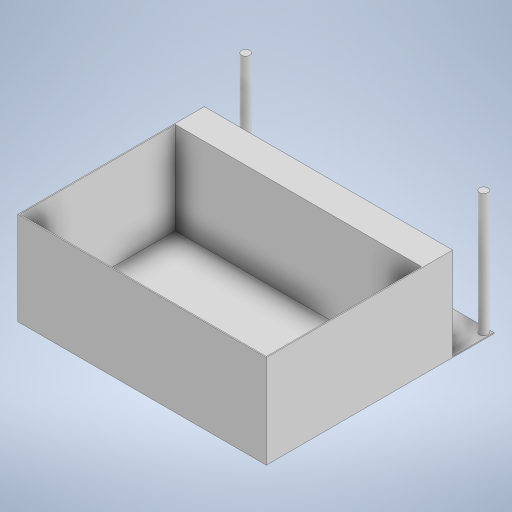
# Autodesk Inventor part: Distanced Top Bin
Saved by Autodesk Inventor 2024 (Build 280153000, 153)
## iProperties
Created: 2024-09-18
Part Number: Distanced Top Bin
Material: Generic
Document SubType Name: Modeling
Designer: srira
Density: 1 g/cm^3
Appearance: Default
Author: srira
Autodesk Inventor part; units mm, degrees
ref_plane "YZ Plane" through (0, 0, 0) normal (1, 0, 0) x (0, 1, 0)
ref_plane "XZ Plane" through (0, 0, 0) normal (0, 1, 0) x (-1, 0, 0)
ref_plane "XY Plane" through (0, 0, 0) normal (0, 0, 1) x (1, 0, 0)
sketch "Sketch1" plane through (0, 0, 0) normal (0, 1, 0) x (-1, 0, 0)
  line L0 (-600, 450) -> (600, 450)
  line L1 (600, 450) -> (600, -450)
  line L2 (600, -450) -> (-600, -450)
  line L3 (-600, -450) -> (-600, 450)
  line L4 (-600, 450) -> (600, -450) construction
  line L5 (600, 450) -> (-600, -450) construction
  line L6 (595, 445) -> (-595, 445)
  line L7 (-595, 445) -> (-595, -305)
  line L8 (-595, -305) -> (595, -305)
  line L9 (595, -305) -> (595, 445)
  point P0 (0, 0)
  dimension "d0" = 1200
  dimension "d1" = 900
  dimension "d2" = 1190
  dimension "d3" = 750
  constraints: 20 end point, 4 parallel, 2 horizontal, 2 midpoint, 2 perpendicular
  measures "d0" distance of L1.end L2.end
  measures "d1" distance of L0.end L1.end
  measures "d2" distance of L8.end L7.end
  measures "d3" distance of L7.end L6.end
extrude "Extrusion1" add sketch "Sketch1" along normal blind 450
ref_plane "Work Plane3" through (0, 0, 0) normal (0, 1, 0) x (1, 0, 0)
sketch "Sketch4" plane through (0, 0, 0) normal (0, 1, 0) x (1, 0, 0)
  line L0 (600, 450) -> (-600, 450) projected
  line L1 (-600, 450) -> (600, 450)
  line L2 (600, 450) -> (600, 650)
  line L3 (600, 650) -> (-600, 650)
  line L4 (-600, 650) -> (-600, 450)
  circle A0 centre (-575, 625) radius 20
  circle A1 centre (575, 625) radius 20
  point P0 (0, 0)
  dimension "d12" = 1200
  dimension "d13" = 200
  dimension "d14" = 40
  dimension "d15" = 40
  constraints: 8 end point, 2 centre point, 2 parallel, 1 horizontal, 1 perpendicular
  measures "d12" distance of L3.end L2.end
  measures "d13" distance of L2.end L1.end
  measures "d14" diameter of A0
  measures "d15" diameter of A1
extrude "Extrusion2" add sketch "Sketch4" along normal blind 600 contours A0 | A1
ref_plane "Work Plane6" through (0, 0, 0) normal (0, 1, 0) x (1, 0, 0)
sketch "Sketch5" plane through (0, 0, 0) normal (0, 1, 0) x (1, 0, 0)
  line L0 (-600, 450) -> (600, 450)
  line L1 (600, 450) -> (600, 650)
  line L2 (600, 650) -> (-600, 650)
  line L3 (-600, 650) -> (-600, 450)
  point P0 (0, 0)
  dimension "d18" = 1200
  dimension "d19" = 200
  constraints: 8 end point, 2 parallel, 1 horizontal, 1 perpendicular
  measures "d18" distance of L2.end L1.end
  measures "d19" distance of L1.end L0.end
extrude "Extrusion3" add sketch "Sketch5" along normal blind 5
ref_plane "Work Plane7" through (0, 0, 0) normal (0, 1, 0) x (1, 0, 0)
sketch "Sketch6" plane through (0, 0, 0) normal (0, 1, 0) x (1, 0, 0)
  line L0 (-595, 305) -> (595, 305) projected
  line L1 (595, -445) -> (-595, -445) projected
  line L2 (595, 305) -> (-595, 305)
  line L3 (-595, 305) -> (-595, -445)
  line L4 (-595, -445) -> (595, -445)
  line L5 (595, -445) -> (595, 305)
  point P0 (0, 0)
  constraints: 8 end point, 2 parallel, 1 horizontal, 1 perpendicular
extrude "Extrusion4" add sketch "Sketch6" along normal blind 5
body "Solid1"
